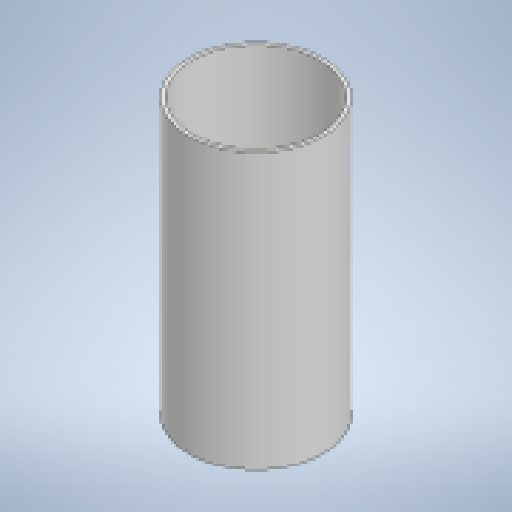
# Autodesk Inventor part: DSB 212 head tube
Saved by Autodesk Inventor 2025 (Build 290162010, 162A)
## iProperties
Created: 2024-12-09
Part Number: DSB 212 head tube
Material: Stainless Steel
Document SubType Name: Modeling
Designer: user
Mass: 1115.89 g
Surface Area: 1404.17 cm^2
Volume: 139.487 cm^3
Density: 8 g/cm^3
Sheet Metal Width: 0,000 mm
Sheet Metal Length: 0,000 mm
Sheet Metal Area: 0,000 mm^2
Appearance: Default
Octaeder_side: 55.919 mm
Octaeder_flange_lenth: 72.500 mm
Author: user
Autodesk Inventor part; units mm, degrees
ref_plane "YZ Plane" through (0, 0, 0) normal (1, 0, 0) x (0, 1, 0)
ref_plane "XZ Plane" through (0, 0, 0) normal (0, 1, 0) x (-1, 0, 0)
ref_plane "XY Plane" through (0, 0, 0) normal (0, 0, 1) x (1, 0, 0)
sketch "Sketch8" plane through (0, 0, 0) normal (0, 0, 1) x (1, 0, 0)
  circle A0 centre (0, 0) radius 38
  circle A1 centre (0, 0) radius 36
  dimension "d46" = 76
  dimension "d47" = 2
  constraints: 2 centre point, 1 coincident
  measures "d46" diameter of A0
  measures "d47" radial gap between concentric circles of A0 A1
extrude "Extrusion2" add sketch "Sketch8" against normal blind 157
equation "\"BendReliefWidth\" = Thickness"
equation "\"BendReliefDepth\" = 0.5 * Thickness"
equation "\"CornerReliefSize\" = 4 * Thickness"
equation "\"MinimumRemnant\" = 2 * Thickness"
equation "\"TransitionRadius\" = BendRadius"
equation "\"JacobiRadiusSize\" = BendRadius"
equation "\"GapSize\" = Thickness"
equation "\"Octaeder_side\" = d41"
equation "\"Octaeder_flange_lenth\" = d42"
equation "\"Thickness\" = 4"
equation "\"BendRadius\" = 6"
equation "\"d41\" = 55.918831"
equation "\"d42\" = 72.5"
body "Solid2"
